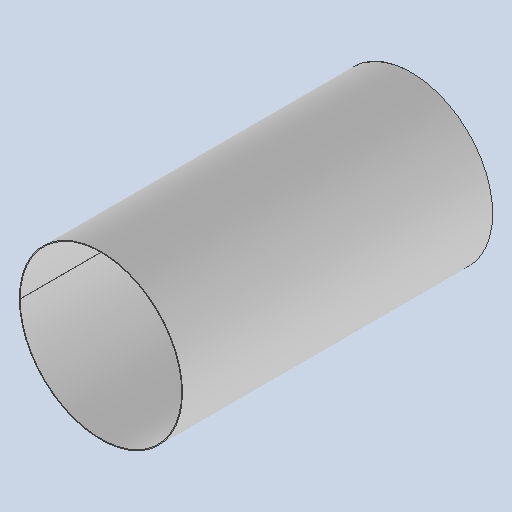
# Autodesk Inventor part: MSC 102 roсket body
Saved by Autodesk Inventor 2025 (Build 290162010, 162A)
## iProperties
Created: 2024-05-19
Part Number: MSC 102 roсket body
Material: Stainless Steel
Document SubType Name: Sheet Metal
Designer: admin
Density: 8 g/cm^3
Flat Pattern Width: 32 cm
Flat Pattern Length: 52.5769 cm
Flat Pattern Area: 1682.46 cm^2
Sheet Metal Rule: Default
Sheet Metal Width: 320,000 mm
Sheet Metal Length: 525,769 mm
Sheet Metal Area: 168246,108 mm^2
Appearance: Default
Stock Number: МОО 102 ракета тело
Mass: 1077.39 g
Surface Area: 3380.39 cm^2
Volume: 134.674 cm^3
Author: admin
Autodesk Inventor part; units mm, degrees
ref_plane "YZ Plane" through (0, 0, 0) normal (1, 0, 0) x (0, 1, 0)
ref_plane "XZ Plane" through (0, 0, 0) normal (0, 1, 0) x (-1, 0, 0)
ref_plane "XY Plane" through (0, 0, 0) normal (0, 0, 1) x (1, 0, 0)
sketch "Sketch1" plane through (0, 0, 0) normal (0, 0, 1) x (1, 0, 0)
  line L0 (0, 0) -> (0, 320)
  line L1 (-83.35, 320) -> (-84.15, 320)
  line L2 (-84.15, 320) -> (-84.15, 0)
  line L3 (-84.15, 0) -> (-83.35, 0)
  line L4 (-83.35, 0) -> (-83.35, 320)
  line L5 (-83.35, 320) -> (-84.15, 0) construction
  line L6 (-84.15, 320) -> (-83.35, 0) construction
  point P0 (-83.75, 160)
  dimension "d0" = 320
  dimension "d1" = 0.8
  dimension "d2" = 168.3
  constraints: 14 end point, 2 midpoint, 2 parallel, 2 point on line, 1 horizontal, 1 perpendicular, 1 vertical
  measures "d0" distance of L0.start L0.end
  measures "d1" distance of L1.start L1.end
  measures "d2" diameter of L2 L0
revolve "Revolution1" add sketch "Sketch1" angle 359.9 about axis through (0, 0, 0) along (0, 1, 0)
equation "\"d1\" = Thickness"
equation "\"BendRadius\" = Thickness"
equation "\"BendReliefWidth\" = Thickness"
equation "\"BendReliefDepth\" = 0.5 * Thickness"
equation "\"CornerReliefSize\" = 4 * Thickness"
equation "\"MinimumRemnant\" = 2 * Thickness"
equation "\"TransitionRadius\" = BendRadius"
equation "\"JacobiRadiusSize\" = BendRadius"
equation "\"GapSize\" = Thickness"
equation "\"Thickness\" = 0.8"
body "Solid1"
